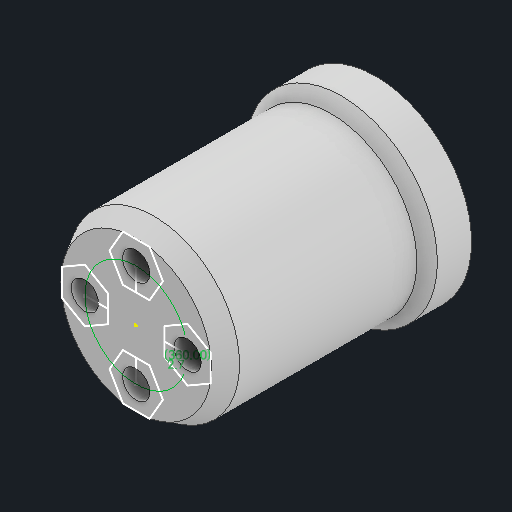
# Autodesk Inventor part: Test_Shaft
Saved by Autodesk Inventor 2025.1 (Build 291241020, 241B)
## iProperties
Created: 2025-07-24
Part Number: Test_Shaft
Material: 일반
Document SubType Name: Modeling
Designer: acalo
Density: 1 g/cm^3
Appearance: 기본값
Author: acalo
Autodesk Inventor part; units mm, degrees
ref_plane "YZ Plane" through (0, 0, 0) normal (1, 0, 0) x (0, 1, 0)
ref_plane "XZ Plane" through (0, 0, 0) normal (0, 1, 0) x (-1, 0, 0)
ref_plane "XY Plane" through (0, 0, 0) normal (0, 0, 1) x (1, 0, 0)
sketch "스케치1" plane through (0, 0, 0) normal (0, 0, 1) x (1, 0, 0)
  circle A0 centre (0, 0) radius 10
  line L0 (0, 0) -> (6, 0)
  line L1 (0, 0) -> (0, 6.1705) construction
  circle A1 centre (6, 0) radius 1.6
  circle A2 centre (-6, 0) radius 1.6
  line L2 (0, 0) -> (0, -6)
  circle A3 centre (0, -6) radius 1.6
  circle A4 centre (0, 6) radius 1.6
  dimension "d0" = 20
  dimension "d1" = 6
  dimension "d2" = 3.2
  dimension "d22" = 6
  dimension "d23" = 3.2
  constraints: 6 end point, 5 centre point, 3 coincident, 2 symmetric about line, 2 vertical, 1 horizontal, 2 other
  measures "d0" diameter of A0
  measures "d1" distance of L0.start L0.end
  measures "d2" diameter of A1
  measures "d22" distance of L0.start L2.end
  measures "d23" diameter of A3
extrude "돌출1" add sketch "스케치1" along normal blind 35
sketch "스케치2" plane through (0, 0, 35) normal (0, 0, 1) x (1, 0, 0)
  line L0 (6, 0) -> (3.3, 0)
  line L1 (3.3, 1.5588) -> (6, 3.1177)
  line L2 (6, 3.1177) -> (8.7, 1.5588)
  line L3 (8.7, 1.5588) -> (8.7, -1.5588)
  line L4 (8.7, -1.5588) -> (6, -3.1177)
  line L5 (6, -3.1177) -> (3.3, -1.5588)
  line L6 (3.3, -1.5588) -> (3.3, 1.5588)
  line L7 (0, 6) -> (0, 3.3)
  line L8 (-1.5588, 3.3) -> (-3.1177, 6)
  line L9 (-3.1177, 6) -> (-1.5588, 8.7)
  line L10 (-1.5588, 8.7) -> (1.5588, 8.7)
  line L11 (1.5588, 8.7) -> (3.1177, 6)
  line L12 (3.1177, 6) -> (1.5588, 3.3)
  line L13 (1.5588, 3.3) -> (-1.5588, 3.3)
  line L14 (-6, 0) -> (-3.3, 0)
  line L15 (-3.3, -1.5588) -> (-6, -3.1177)
  line L16 (-6, -3.1177) -> (-8.7, -1.5588)
  line L17 (-8.7, -1.5588) -> (-8.7, 1.5588)
  line L18 (-8.7, 1.5588) -> (-6, 3.1177)
  line L19 (-6, 3.1177) -> (-3.3, 1.5588)
  line L20 (-3.3, 1.5588) -> (-3.3, -1.5588)
  line L21 (0, -6) -> (0, -3.3)
  line L22 (1.5588, -3.3) -> (3.1177, -6)
  line L23 (3.1177, -6) -> (1.5588, -8.7)
  line L24 (1.5588, -8.7) -> (-1.5588, -8.7)
  line L25 (-1.5588, -8.7) -> (-3.1177, -6)
  line L26 (-3.1177, -6) -> (-1.5588, -3.3)
  line L27 (-1.5588, -3.3) -> (1.5588, -3.3)
  point P0 (0, 0)
  point P1 (0, 6)
  point P2 (0, -6)
  dimension "d24" = 2.7
  dimension "d27" = 360
  constraints: 56 end point, 4 coincident, 1 horizontal, 1 midpoint, 78 other
  measures "d24" distance of L0.start L0.end
sketch "스케치3" plane through (0, 0, 0) normal (0, 0, -1) x (-1, 0, 0)
  circle A0 centre (0, 0) radius 10 projected
  circle A1 centre (-6, 0) radius 1.6 projected
  circle A2 centre (6, 0) radius 1.6 projected
extrude "돌출3" cut sketch "스케치3" against normal blind 7
sketch "스케치4" plane through (0, 0, 7) normal (0, 0, -1) x (-1, 0, 0)
  circle A0 centre (0, 0) radius 10 projected
  circle A1 centre (0, 0) radius 11.2
  dimension "d13" = 1.2
  constraints: 1 centre point
  measures "d13" radial gap between concentric circles of A0 A1
extrude "돌출4" add sketch "스케치4" against normal blind 4
chamfer "모따기2" distance 1.2 angle 45 1 edges at (-10, 0, 11)
chamfer "모따기3" distance 1.2 angle 60 1 edges at (-10, 0, 35) measured on face at (-9.5, 0, 35)
